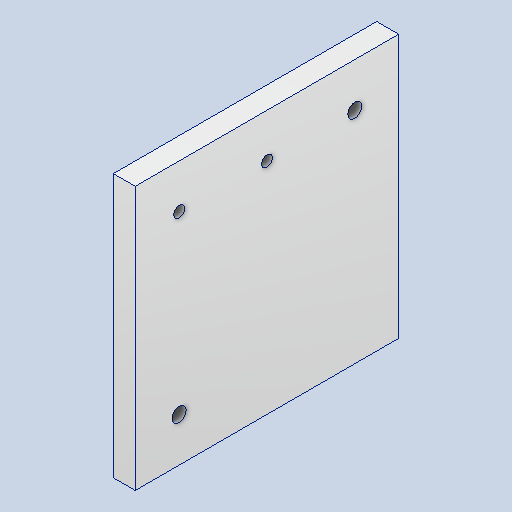
# Autodesk Inventor part: base_weel-v3-Plate-8
Saved by Autodesk Inventor 2025.2 (Build 292293000, 293)
## iProperties
Created: 2025-04-05
Part Number: base_weel-v3-Plate-8
Material: アルミニウム 6061
Document SubType Name: Modeling
Designer: haruy
Density: 2.7 g/cm^3
Appearance: アルミニウム - フラット
Author: haruy
Autodesk Inventor part; units mm, degrees
ref_plane "YZ Plane" through (0, 0, 0) normal (1, 0, 0) x (0, 1, 0)
ref_plane "XZ Plane" through (0, 0, 0) normal (0, 1, 0) x (-1, 0, 0)
ref_plane "XY Plane" through (0, 0, 0) normal (0, 0, 1) x (1, 0, 0)
derived "base_weel-v3-ASP-Base.ipt"
sketch "スケッチ9" plane through (0, -300, -190) normal (1, 0, 0) x (0, 0, -1)
  line L0 (-215, 15) -> (-165, 15) projected
  line L1 (-165, 15) -> (-165, -35) projected
  line L2 (-165, -35) -> (-215, -35) projected
  line L3 (-215, -35) -> (-215, 15) projected
  circle A0 centre (-190, -10) radius 22 projected
  line L4 (-212, -10) -> (-168, -10) projected
  line L5 (-380, 0) -> (0, 0) projected
  line L6 (-268.5, 20) -> (-268.5, 241.5) projected
  line L7 (-220, 20) -> (-160, 20) projected
  line L8 (-160, 20) -> (-160, -40) projected
  line L9 (-160, -40) -> (-220, -40) projected
  line L10 (-220, -40) -> (-220, 20) projected
  circle A1 centre (-170, 10) radius 1.6 projected
  line L11 (0, 20) -> (-380, 20) projected
  circle A2 centre (-210, 10) radius 1.25 projected
  circle A3 centre (-190, 10) radius 1.25 projected
  circle A4 centre (-210, -30) radius 1.6
  point P0 (-190, 300)
  dimension "d1" = 3.2
  dimension "d2" = 5
  dimension "d3" = 5
  constraints: 1 centre point
  measures "d1" diameter of A4
  measures "d2" distance from line of A4.centre L2
  measures "d3" distance from line of A4.centre L3
extrude "押し出し1" add sketch "スケッチ9" against normal blind 5
